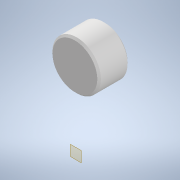
# Autodesk Inventor part: ciezarek1
Saved by Autodesk Inventor 2021 (Build 250183000, 183)
## iProperties
Created: 2021-06-18
Part Number: ciezarek1
Material: Stal, miękka
Document SubType Name: Modeling
Designer: Wojciech Wołczek
Density: 7.85 g/cm^3
Appearance: Częściowo polerowana
Author: Wojciech Wołczek
Autodesk Inventor part; units mm, degrees
ref_plane "YZ Plane" through (0, 0, 0) normal (1, 0, 0) x (0, 1, 0)
ref_plane "XZ Plane" through (0, 0, 0) normal (0, 1, 0) x (-1, 0, 0)
ref_plane "XY Plane" through (0, 0, 0) normal (0, 0, 1) x (1, 0, 0)
ref_plane "Płaszczyzna konstrukcyjna1" through (201.2988, -605.9727, -25) normal (0, 0, 1) x (0.0012, 1, 0)
sketch "Szkic1" plane through (201.2988, -605.9727, -25) normal (0, 0, 1) x (0.0012, 1, 0)
  circle A0 centre (123.9991, 1.6821) radius 10
  circle A1 centre (123.9991, 1.6821) radius 40
  ellipse E0 centre (181.2886, 11.8263) end of major axis (181.2615, 21.8263) minor radius 10 projected
  point P0 (605.7397, 201.9988)
  dimension "d0" = 80
  constraints: 2 centre point, 1 coincident, 2 other
  measures "d0" diameter of A1
extrude "Wyciągnięcie proste1" add sketch "Szkic1" against normal blind 50 contours A0 | A1
chamfer "Faza1" distance 3 angle 45 2 edges at (199.7137, -521.9717, -25) (199.7137, -521.9717, -75)
